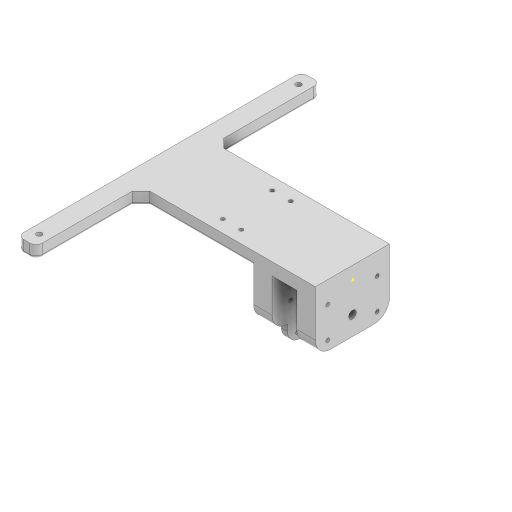
# Autodesk Inventor part: PanelBarcket
Saved by Autodesk Inventor 2023 (Build 270158000, 158)
## iProperties
Created: 2023-10-18
Part Number: PanelBarcket
Material: Generic
Document SubType Name: Modeling
Designer: MVeszpremi
Density: 1 g/cm^3
Appearance: Default
Author: MVeszpremi
Autodesk Inventor part; units mm, degrees
ref_plane "YZ Plane" through (0, 0, 0) normal (1, 0, 0) x (0, 1, 0)
ref_plane "XZ Plane" through (0, 0, 0) normal (0, 1, 0) x (-1, 0, 0)
ref_plane "XY Plane" through (0, 0, 0) normal (0, 0, 1) x (1, 0, 0)
sketch "Sketch1" plane through (0, 0, 0) normal (0, 1, 0) x (-1, 0, 0)
  line L0 (-148.75, 105) -> (148.75, 105)
  line L1 (148.75, 105) -> (148.75, -105)
  line L2 (148.75, -105) -> (-148.75, -105)
  line L3 (-148.75, -105) -> (-148.75, 105)
  line L4 (-148.75, 105) -> (148.75, -105) construction
  line L5 (148.75, 105) -> (-148.75, -105) construction
  circle A0 centre (148.75, -105) radius 2.15
  circle A1 centre (148.75, 105) radius 2.15
  line L6 (156.25, 115) -> (141.25, 115)
  line L7 (141.25, 115) -> (141.25, -115)
  line L8 (141.25, -115) -> (156.25, -115)
  line L9 (156.25, -115) -> (156.25, 115)
  line L10 (156.25, 115) -> (141.25, -115) construction
  line L11 (141.25, 115) -> (156.25, -115) construction
  line L12 (141.25, -30) -> (0, -30)
  line L13 (0, -30) -> (0, 30)
  line L14 (0, 30) -> (141.25, 30)
  line L15 (141.25, 30) -> (141.25, -30)
  point P0 (0, 0)
  point P1 (148.75, 0)
  point P2 (141.25, 30)
  dimension "d0" = 297.5
  dimension "d1" = 210
  dimension "d2" = 4.3
  dimension "d3" = 4.3
  dimension "d4" = 15
  dimension "d5" = 230
  dimension "d6" = 30
  dimension "d7" = 30
  constraints: 32 end point, 6 parallel, 5 midpoint, 3 horizontal, 3 perpendicular, 2 centre point, 2 coincident, 1 point on line
  measures "d0" distance of L1.end L2.end
  measures "d1" distance of L0.end L1.end
  measures "d2" diameter of A0
  measures "d3" diameter of A1
  measures "d4" distance of L7.end L8.end
  measures "d5" distance of L8.end L6.start
  measures "d6" distance from line of point (148.75, 0) L12
  measures "d7" distance from line of L14 point (148.75, 0)
extrude "Extrusion1" add sketch "Sketch1" along normal blind 10 contours L7 L6 L9 L8 L2 A0 L1 A1 L0 | L0 A1 L1 A0 L2 L7 | L7 L12 L13 L14
sketch "Sketch2" plane through (0, 0, 0) normal (0, -1, 0) x (1, 0, 0)
  circle A0 centre (-148.75, 105) radius 2.15 projected
  circle A1 centre (-148.75, 105) radius 4.5
  circle A2 centre (-148.75, -105) radius 2.15 projected
  circle A3 centre (-148.75, -105) radius 4.5
  point P0 (0, 0)
  dimension "d10" = 9
  dimension "d11" = 9
  constraints: 2 centre point, 2 coincident
  measures "d10" diameter of A1
  measures "d11" diameter of A3
extrude "Extrusion2" cut sketch "Sketch2" against normal blind 5
sketch "Sketch5" plane through (0, 10, 0) normal (0, 1, 0) x (1, 0, 0)
  line L0 (0, -30) -> (0, 30) projected
  line L1 (-141.25, -30) -> (0, -30) projected
  line L2 (0, 30) -> (-15, 30)
  line L3 (-15, 30) -> (-15, -30)
  line L4 (-15, -30) -> (0, -30)
  line L5 (0, -30) -> (0, 30)
  point P0 (0, 0)
  dimension "d27" = 15
  constraints: 8 end point, 2 parallel, 1 horizontal, 1 perpendicular, 1 point on line
  measures "d27" distance between parallel lines of L0 L3
extrude "Extrusion5" add sketch "Sketch5" against normal blind 50
sketch "Sketch6" plane through (0, 10, 30) normal (1, 0, 0) x (0, 0, -1)
  circle A0 centre (30, -34.5) radius 8.125
  circle A1 centre (30, -34.5) radius 3
  point P0 (30, -10)
  dimension "d30" = 24.5
  dimension "d31" = 16.25
  dimension "d32" = 6
  constraints: 2 centre point, 1 coincident
  measures "d30" distance of A0.centre point (30, -10)
  measures "d31" diameter of A0
  measures "d32" diameter of A1
extrude "Extrusion7" cut sketch "Sketch6" against normal blind 15 contours A1
sketch "Sketch7" plane through (0, 10, 30) normal (1, 0, 0) x (0, 0, -1)
  line L0 (10, -17.5) -> (50, -17.5)
  line L1 (50, -17.5) -> (50, -42.5)
  line L2 (50, -42.5) -> (10, -42.5)
  line L3 (10, -42.5) -> (10, -17.5)
  circle A0 centre (10, -17.5) radius 1.5
  circle A1 centre (50, -17.5) radius 1.5
  circle A2 centre (50, -42.5) radius 1.5
  circle A3 centre (10, -42.5) radius 1.5
  point P0 (30, -10)
  dimension "d37" = 40
  dimension "d38" = 25
  dimension "d39" = 20
  dimension "d40" = 7.5
  dimension "d41" = 3
  dimension "d42" = 3
  dimension "d43" = 3
  dimension "d44" = 3
  constraints: 8 end point, 4 centre point, 4 coincident, 2 parallel, 1 horizontal, 1 perpendicular
  measures "d37" distance of L0.start L0.end
  measures "d38" distance of L2.end L0.start
  measures "d39" distance from line of point (30, -10) L3
  measures "d40" distance from line of point (30, -10) L0
  measures "d41" diameter of A0
  measures "d42" diameter of A1
  measures "d43" diameter of A2
  measures "d44" diameter of A3
extrude "Extrusion8" cut sketch "Sketch7" against normal blind 15 contours L3 A0 L0 | L0 A0 L3 | A1 L1 L0 | L0 L1 A1 | A3 L2 L3 | L3 L2 A3 | A2 L2 L1 | L1 L2 A2
sketch "Sketch8" plane through (0, 0, 0) normal (0, -1, 0) x (1, 0, 0)
  point P0 (0, 0)
sketch "Sketch9" plane through (0, 0, 0) normal (0, -1, 0) x (1, 0, 0)
  line L0 (-141.25, 30) -> (-15, 30) projected
  line L1 (-15, -30) -> (-141.25, -30) projected
  line L2 (-50, 30) -> (-35, 30)
  line L3 (-35, 30) -> (-35, -30)
  line L4 (-35, -30) -> (-50, -30)
  line L5 (-50, -30) -> (-50, 30)
  line L6 (-15, 30) -> (-15, -30) projected
  point P0 (0, 0)
  point P1 (-35, 30)
  dimension "d47" = 15
  dimension "d48" = 20
  constraints: 8 end point, 2 parallel, 2 point on line, 1 horizontal, 1 perpendicular
  measures "d47" distance between parallel lines of L5 L3
  measures "d48" distance between parallel lines of L6 L3
extrude "Extrusion9" add sketch "Sketch9" along normal up to surface (40 mm away) contours L0 L3 L1 L5
sketch "Sketch10" plane through (-50, 0, 40) normal (1, 0, 0) x (0, 0, -1)
  circle A0 centre (40, -24.5) radius 3 projected
  circle A1 centre (40, -24.5) radius 8.125
  circle A2 centre (55, -24.5) radius 1.5
  circle A3 centre (25, -24.5) radius 1.5
  point P0 (40, 0)
  dimension "d51" = 16.25
  dimension "d52" = 3
  dimension "d53" = 3
  dimension "d54" = 15
  dimension "d55" = 15
  constraints: 3 centre point, 2 horizontal alignment, 1 coincident
  measures "d51" diameter of A1
  measures "d52" diameter of A2
  measures "d53" diameter of A3
  measures "d54" distance of A2.centre A1.centre
  measures "d55" distance of A3.centre A1.centre
extrude "Extrusion10" cut sketch "Sketch10" along normal blind 15 contours A0 | A2 | A3
extrude "Extrusion11" cut sketch "Sketch10" along normal blind 7.5 contours A1
sketch "Sketch11" plane through (-50, 0, -30) normal (-1, 0, 0) x (0, 0, 1)
  line L0 (49.5, -33.5) -> (10.5, -33.5)
  line L1 (10.5, -33.5) -> (10.5, -15.5)
  line L2 (10.5, -15.5) -> (49.5, -15.5)
  line L3 (49.5, -15.5) -> (49.5, -33.5)
  circle A0 centre (30, -24.5) radius 3 projected
  line L4 (49.5, -33.5) -> (10.5, -15.5) construction
  line L5 (10.5, -33.5) -> (49.5, -15.5) construction
  point P0 (30, 0)
  dimension "d60" = 18
  dimension "d61" = 39
  constraints: 12 end point, 2 midpoint, 2 parallel, 1 horizontal, 1 perpendicular
  measures "d60" distance of L2.end L0.start
  measures "d61" distance of L0.start L0.end
extrude "Extrusion12" cut sketch "Sketch11" against normal blind 2.5
fillet "Fillet1" radius 12.5 4 edges at (-7.5, -40, -30) (-42.5, -40, -30) (-42.5, -40, 30) (-7.5, -40, 30)
chamfer "Chamfer1" distance 7 angle 45 2 edges at (-141.25, 5, -30) (-141.25, 5, 30)
fillet "Fillet2" radius 2 10 edges at (-92.125, 0, 30) (-141.25, 0, 76) (-137.75, 0, 33.5) (-134.25, 5, -30) (-137.75, 0, -33.5) (-92.125, 0, -30) (-141.25, 0, -76) (-148.75, 0, -115) (-156.25, 0, 0) (-148.75, 0, 115)
fillet "Fillet3" radius 5 8 edges at (-141.8358, 0.5858, 114.4142) (-141.25, 6, 115) (-155.6642, 0.5858, -114.4142) (-156.25, 6, -115) (-141.8358, 0.5858, -114.4142) (-141.25, 6, -115) (-155.6642, 0.5858, 114.4142) (-156.25, 6, 115)
sketch "Sketch12" plane through (0, 0, 0) normal (0, -1, 0) x (1, 0, 0)
  line L0 (-85, 20) -> (-70, 20)
  line L1 (-70, 20) -> (-70, -20)
  line L2 (-70, -20) -> (-85, -20)
  line L3 (-85, -20) -> (-85, 20)
  line L4 (-50, -17.5) -> (-50, 17.5) projected
  circle A0 centre (-85, 20) radius 1.5
  circle A1 centre (-70, 20) radius 1.5
  circle A2 centre (-70, -20) radius 1.5
  circle A3 centre (-85, -20) radius 1.5
  point P0 (0, 0)
  point P1 (-50, 0)
  point P2 (-50, 0)
  point P3 (-77.5, -20)
  dimension "d70" = 20
  dimension "d71" = 20
  dimension "d72" = 20
  dimension "d73" = 15
  dimension "d74" = 3
  dimension "d75" = 3
  dimension "d76" = 3
  dimension "d77" = 3
  constraints: 8 end point, 4 centre point, 4 coincident, 3 midpoint, 2 parallel, 1 horizontal, 1 perpendicular
  measures "d70" distance from line of L0 point (-50, 0)
  measures "d71" vertical distance of point (-50, 0) point (-77.5, -20)
  measures "d72" distance between parallel lines of L4 L1
  measures "d73" distance of L0.start L0.end
  measures "d74" diameter of A0
  measures "d75" diameter of A1
  measures "d76" diameter of A3
  measures "d77" diameter of A2
extrude "Extrusion13" cut sketch "Sketch12" against normal blind 20 contours L3 A0 L0 | L0 A0 L3 | A1 L1 L0 | L0 L1 A1 | A3 L2 L3 | L3 L2 A3 | A2 L2 L1 | L1 L2 A2
sketch "Sketch13" plane through (-50, -40, 17.5) normal (0, -1, 0) x (1, 0, 0)
  line L0 (0, 0) -> (15, 0) projected
  line L1 (15, -35) -> (0, -35) projected
  line L2 (15, 0) -> (10, 0)
  line L3 (10, 0) -> (10, -35)
  line L4 (10, -35) -> (15, -35)
  line L5 (15, -35) -> (15, 0)
  point P0 (50, -17.5)
  point P1 (10, 0)
  dimension "d80" = 5
  constraints: 8 end point, 2 parallel, 1 horizontal, 1 perpendicular, 1 point on line
  measures "d80" distance between parallel lines of L5 L3
extrude "Extrusion14" add sketch "Sketch13" along normal blind 15
sketch "Sketch14" plane through (-40, -40, -17.5) normal (-1, 0, 0) x (0, 0, 1)
  circle A0 centre (27, -9.5) radius 1.5
  circle A1 centre (8, -9.5) radius 1.5
  circle A2 centre (17.5, 15.5) radius 3 projected
  point P0 (17.5, 40)
  dimension "d83" = 9.5
  dimension "d84" = 9.5
  dimension "d85" = 3
  dimension "d86" = 3
  dimension "d94" = 25
  constraints: 2 centre point, 1 horizontal alignment
  measures "d83" horizontal distance of A0.centre A2.centre
  measures "d84" horizontal distance of A2.centre A1.centre
  measures "d85" diameter of A0
  measures "d86" diameter of A1
  measures "d94" vertical distance of A2.centre A0.centre
extrude "Extrusion15" cut sketch "Sketch14" against normal blind 15 contours A0 | A1
sketch "Sketch17" plane through (-40, -40, -17.5) normal (-1, 0, 0) x (0, 0, 1)
  line L0 (0, -15) -> (35, -15) projected
  line L1 (21.5, -15) -> (12, -15)
  line L2 (12, -15) -> (12, -6)
  line L3 (12, -6) -> (21.5, -6)
  line L4 (21.5, -6) -> (21.5, -15)
  circle A0 centre (27, -9.5) radius 1.5 projected
  circle A1 centre (8, -9.5) radius 1.5 projected
  line L5 (21.5, -13) -> (12, -13)
  point P0 (17.5, 40)
  point P1 (17.5, -15)
  dimension "d89" = 4
  dimension "d90" = 4
  dimension "d91" = 9
  dimension "d95" = 2
  constraints: 10 end point, 3 point on line, 2 parallel, 2 perpendicular, 1 horizontal, 1 midpoint
  measures "d89" distance edge to line of A0 L4
  measures "d90" distance from line of A1.centre L2
  measures "d91" distance of L3.end L1.start
  measures "d95" distance from line of point (17.5, -15) L5
extrude "Extrusion16" cut sketch "Sketch17" against normal blind 4 contours L2 L3 L4 L5
fillet "Fillet4" radius 10 2 edges at (-37.5, -55, 17.5) (-37.5, -55, -17.5)
body "Solid1"
